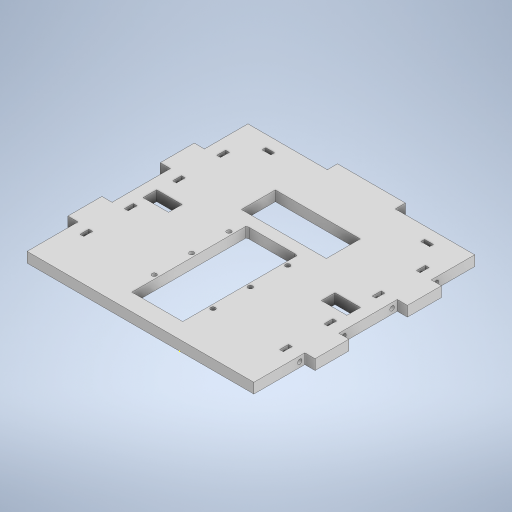
# Autodesk Inventor part: frame_upper1
Saved by Autodesk Inventor 2024 (Build 280153000, 153)
## iProperties
Created: 2024-09-07
Part Number: frame_upper1
Material: 일반
Document SubType Name: Modeling
Designer: jmha0
Density: 1 g/cm^3
Appearance: 기본값
Mass: 87.8648 g
Surface Area: 361.939 cm^2
Volume: 87.8648 cm^3
Author: jmha0
Autodesk Inventor part; units mm, degrees
(part 1 of 2)
ref_plane "YZ Plane" through (0, 0, 0) normal (1, 0, 0) x (0, 1, 0)
ref_plane "XZ Plane" through (0, 0, 0) normal (0, 1, 0) x (-1, 0, 0)
ref_plane "XY Plane" through (0, 0, 0) normal (0, 0, 1) x (1, 0, 0)
sketch "스케치1" plane through (0, 0, 0) normal (0, 1, 0) x (-1, 0, 0)
  line L0 (-51.929, 23.5866) -> (-51.929, -10.2551)
  line L1 (-51.929, -10.2551) -> (-45.929, -10.2551)
  line L2 (-45.929, -10.2551) -> (-45.929, -50.2551)
  line L3 (-45.929, -50.2551) -> (-51.929, -50.2551)
  line L4 (-51.929, -50.2551) -> (-51.929, -112.0968)
  line L5 (-51.929, -112.0968) -> (97.1074, -112.0968)
  line L6 (97.1074, -112.0968) -> (97.1074, -50.2551)
  line L7 (97.1074, -50.2551) -> (92.3803, -50.2551)
  line L8 (92.3803, -50.2551) -> (92.3803, -10.2551)
  line L9 (92.3803, -10.2551) -> (97.7439, -10.2551)
  line L10 (97.7439, -10.2551) -> (97.7439, 23.5866)
  line L11 (-51.929, 23.5866) -> (97.7439, 23.5866)
  line L12 (57.1074, -50.2551) -> (51.1074, -50.2551)
  line L13 (51.1074, -50.2551) -> (51.1074, -10.2551)
  line L14 (51.1074, -10.2551) -> (57.1074, -10.2551)
  line L15 (57.1074, -10.2551) -> (57.1074, -50.2551)
  line L16 (-5.2926, -50.2551) -> (-11.2926, -50.2551)
  line L17 (-11.2926, -50.2551) -> (-11.2926, -10.2551)
  line L18 (-11.2926, -10.2551) -> (-5.2926, -10.2551)
  line L19 (-5.2926, -10.2551) -> (-5.2926, -50.2551)
  circle A0 centre (40.2074, -56.8968) radius 1.45
  circle A1 centre (5.6074, -56.8968) radius 1.45
  circle A2 centre (40.2074, -34.8968) radius 1.45
  circle A3 centre (5.6074, -34.8968) radius 1.45
  circle A4 centre (40.2074, -12.8968) radius 1.45
  circle A5 centre (5.6074, -12.8968) radius 1.45
  line L20 (37.6074, 2.5866) -> (37.6074, -73.0968)
  line L21 (37.6074, -73.0968) -> (8.2074, -73.0968)
  line L22 (8.2074, -73.0968) -> (8.2074, 2.5866)
  line L23 (8.2074, 2.5866) -> (37.6074, 2.5866)
  line L24 (89.8574, 258.2156) -> (-43.6426, 258.2156)
  line L25 (-43.6426, 128.2156) -> (89.8574, 128.2156)
  arc A6 (3.3266, -10.6333) -> (2.8074, -12.3202) centre (5.8074, -12.3202) ccw
  line L26 (2.8074, -56.5734) -> (2.8074, -12.3202)
  arc A7 (2.8074, -56.5734) -> (3.3266, -58.2604) centre (5.8074, -56.5734) ccw
  line L27 (7.0145, -63.6837) -> (3.3266, -58.2604)
  arc A8 (7.0145, -63.6837) -> (9.4953, -64.9968) centre (9.4953, -61.9968) ccw
  line L28 (36.3195, -64.9968) -> (9.4953, -64.9968)
  arc A9 (36.3195, -64.9968) -> (38.8003, -63.6837) centre (36.3195, -61.9968) ccw
  line L29 (42.4882, -58.2604) -> (38.8003, -63.6837)
  arc A10 (42.4882, -58.2604) -> (43.0074, -56.5734) centre (40.0074, -56.5734) ccw
  line L30 (43.0074, -12.3202) -> (43.0074, -56.5734)
  arc A11 (43.0074, -12.3202) -> (42.4882, -10.6333) centre (40.0074, -12.3202) ccw
  line L31 (38.5027, -4.7722) -> (42.4882, -10.6333)
  arc A12 (38.5027, -4.7722) -> (36.8488, -3.8968) centre (36.8488, -5.8968) ccw
  line L32 (30.5574, -3.8968) -> (36.8488, -3.8968)
  arc A13 (32.0574, -5.3968) -> (30.5574, -3.8968) centre (30.5574, -5.3968) ccw
  line L33 (32.0574, -5.3968) -> (32.0574, -6.8968)
  arc A14 (32.0574, -6.8968) -> (34.4074, -9.2468) centre (34.4074, -6.8968) ccw
  line L34 (34.4074, -9.2468) -> (36.4074, -9.2468)
  arc A15 (37.4074, -10.2468) -> (36.4074, -9.2468) centre (36.4074, -10.2468) ccw
  line L35 (37.4074, -10.2468) -> (37.4074, -53.0468)
  arc A16 (36.4074, -54.0468) -> (37.4074, -53.0468) centre (36.4074, -53.0468) ccw
  line L36 (36.4074, -54.0468) -> (34.4074, -54.0468)
  arc A17 (34.4074, -54.0468) -> (32.0574, -56.3968) centre (34.4074, -56.3968) ccw
  line L37 (32.0574, -56.3968) -> (32.0574, -58.3968)
  arc A18 (31.0574, -59.3968) -> (32.0574, -58.3968) centre (31.0574, -58.3968) ccw
  line L38 (31.0574, -59.3968) -> (14.7574, -59.3968)
  arc A19 (13.7574, -58.3968) -> (14.7574, -59.3968) centre (14.7574, -58.3968) ccw
  line L39 (13.7574, -58.3968) -> (13.7574, -56.3968)
  arc A20 (13.7574, -56.3968) -> (11.4074, -54.0468) centre (11.4074, -56.3968) ccw
  line L40 (11.4074, -54.0468) -> (9.4074, -54.0468)
  arc A21 (8.4074, -53.0468) -> (9.4074, -54.0468) centre (9.4074, -53.0468) ccw
  line L41 (8.4074, -53.0468) -> (8.4074, -10.2468)
  arc A22 (9.4074, -9.2468) -> (8.4074, -10.2468) centre (9.4074, -10.2468) ccw
  line L42 (9.4074, -9.2468) -> (11.4074, -9.2468)
  arc A23 (11.4074, -9.2468) -> (13.7574, -6.8968) centre (11.4074, -6.8968) ccw
  line L43 (13.7574, -6.8968) -> (13.7574, -5.3968)
  arc A24 (15.2574, -3.8968) -> (13.7574, -5.3968) centre (15.2574, -5.3968) ccw
  line L44 (8.966, -3.8968) -> (15.2574, -3.8968)
  arc A25 (8.966, -3.8968) -> (7.3121, -4.7722) centre (8.966, -5.8968) ccw
  line L45 (3.3266, -10.6333) -> (7.3121, -4.7722)
  circle A26 centre (40.2074, -12.8968) radius 1.35
  circle A27 centre (40.2074, -34.8968) radius 1.35
  circle A28 centre (33.9074, -62.1968) radius 1.35
  circle A29 centre (5.6074, -12.8968) radius 1.35
  circle A30 centre (5.6074, -34.8968) radius 1.35
  circle A31 centre (11.9074, -62.1968) radius 1.35
  circle A32 centre (40.2074, -56.8968) radius 1.35
  circle A33 centre (5.6074, -56.8968) radius 1.35
  circle A34 centre (22.9074, -16.8968) radius 13.8
  circle A35 centre (22.9074, -27.8968) radius 1.2813
  circle A36 centre (30.6856, -24.675) radius 1.2813
  circle A37 centre (33.9074, -16.8968) radius 1.2813
  circle A38 centre (30.6856, -9.1186) radius 1.2813
  circle A39 centre (22.9074, -5.8968) radius 1.2813
  circle A40 centre (15.1292, -9.1186) radius 1.2813
  circle A41 centre (22.9074, -16.8968) radius 13.8
  circle A42 centre (22.9074, -16.8968) radius 7.2
  circle A43 centre (22.9074, -27.8968) radius 1.2813
  circle A44 centre (15.1292, -24.675) radius 1.2813
  circle A45 centre (11.9074, -16.8968) radius 1.2813
  circle A46 centre (15.1292, -9.1186) radius 1.2813
  circle A47 centre (22.9074, -5.8968) radius 1.2813
  circle A48 centre (30.6856, -9.1186) radius 1.2813
  circle A49 centre (33.9074, -16.8968) radius 1.2813
  circle A50 centre (30.6856, -24.675) radius 1.2813
  line L46 (23.1074, 258.2156) -> (23.1074, 238.2156)
  line L47 (23.2304, 248.2156) -> (38.2304, 248.2156)
  line L48 (38.2304, 248.2156) -> (8.2304, 248.2156)
  line L49 (8.2304, 248.2156) -> (8.2304, 173.2156)
  line L50 (8.2304, 173.2156) -> (38.2304, 173.2156)
  line L51 (38.2304, 173.2156) -> (38.2304, 248.2156)
  arc A51 (3.6496, 234.9792) -> (3.1304, 233.2922) centre (6.1304, 233.2922) ccw
  line L52 (3.1304, 189.039) -> (3.1304, 233.2922)
  arc A52 (3.1304, 189.039) -> (3.6496, 187.352) centre (6.1304, 189.039) ccw
  line L53 (7.3375, 181.9287) -> (3.6496, 187.352)
  arc A53 (7.3375, 181.9287) -> (9.8183, 180.6156) centre (9.8183, 183.6156) ccw
  line L54 (36.6425, 180.6156) -> (9.8183, 180.6156)
  arc A54 (36.6425, 180.6156) -> (39.1233, 181.9287) centre (36.6425, 183.6156) ccw
  line L55 (42.8112, 187.352) -> (39.1233, 181.9287)
  arc A55 (42.8112, 187.352) -> (43.3304, 189.039) centre (40.3304, 189.039) ccw
  line L56 (43.3304, 233.2922) -> (43.3304, 189.039)
  arc A56 (43.3304, 233.2922) -> (42.8112, 234.9792) centre (40.3304, 233.2922) ccw
  line L57 (38.8256, 240.8402) -> (42.8112, 234.9792)
  arc A57 (38.8256, 240.8402) -> (37.1718, 241.7156) centre (37.1718, 239.7156) ccw
  line L58 (30.8804, 241.7156) -> (37.1718, 241.7156)
  arc A58 (37.7304, 235.3656) -> (36.7304, 236.3656) centre (36.7304, 235.3656) ccw
  arc A59 (36.7304, 191.5656) -> (37.7304, 192.5656) centre (36.7304, 192.5656) ccw
  arc A60 (8.7304, 192.5656) -> (9.7304, 191.5656) centre (9.7304, 192.5656) ccw
  arc A61 (9.7304, 236.3656) -> (8.7304, 235.3656) centre (9.7304, 235.3656) ccw
  arc A62 (9.289, 241.7156) -> (7.6351, 240.8402) centre (9.289, 239.7156) ccw
  line L59 (3.6496, 234.9792) -> (7.6351, 240.8402)
  circle A63 centre (40.5304, 232.7156) radius 1.45
  circle A64 centre (40.5304, 210.7156) radius 1.45
  circle A65 centre (40.5304, 188.7156) radius 1.45
  circle A66 centre (5.9304, 188.7156) radius 1.45
  circle A67 centre (5.9304, 210.7156) radius 1.45
  circle A68 centre (5.9304, 232.7156) radius 1.45
  line L60 (41.9804, 210.7156) -> (49.8574, 210.7156)
  line L61 (89.8574, 180.7156) -> (89.8574, 220.7156)
  line L62 (-43.6426, 180.7156) -> (-43.6426, 220.7156)
  line L63 (-43.6426, 258.2156) -> (-43.6426, 128.2156)
  line L64 (89.8574, 128.2156) -> (89.8574, 258.2156)
  line L65 (8.2304, 258.2156) -> (8.2304, 248.2156)
  circle A69 centre (40.5304, 188.7156) radius 1.35
  circle A70 centre (40.5304, 210.7156) radius 1.35
  circle A71 centre (40.5304, 232.7156) radius 1.35
  circle A72 centre (5.9304, 232.7156) radius 1.35
  circle A73 centre (5.9304, 210.7156) radius 1.35
  circle A74 centre (5.9304, 188.7156) radius 1.35
  point P0 (0, 0)
  point P1 (54.2167, -116.1391)
  point P2 (22.9074, 23.5866)
  point P3 (22.9074, -16.8968)
  point P4 (38.2304, 181.0703)
  point P5 (8.2304, 181.0703)
  point P6 (8.2304, 241.4125)
  point P7 (38.2304, 241.4125)
  dimension "d0" = 149.0364
  dimension "d1" = 135.6834
  dimension "d4" = 21
  dimension "d5" = 20
  dimension "d6" = 29.4
  dimension "d7" = 75.6834
  dimension "d8" = 15
  dimension "d9" = 30
  dimension "d17" = 40
  dimension "d18" = 6
  dimension "d36" = 130
  dimension "d37" = 133.5
  dimension "d95" = 0.1
  dimension "d96" = 0.1
  dimension "d97" = 0.1
  dimension "d98" = 0.1
  dimension "d99" = 0.1
  dimension "d100" = 0.1
  constraints: 132 end point, 75 centre point, 64 point on circle, 3 horizontal, 3 parallel, 2 midpoint, 2 perpendicular, 2 vertical, 1 point on line
  measures "d0" distance between parallel lines of L6 L4
  measures "d1" distance between parallel lines of L5 L11
  measures "d4" distance from line of point (22.907, 23.587) L23
  measures "d5" distance of L46.end L46.start
  measures "d6" distance of L23.start L23.end
  measures "d7" distance of L23.end L21.start
  measures "d8" distance of L47.start L47.end
  measures "d9" distance of L50.end L49.end
  measures "d17" distance of L14.end L12.start
  measures "d18" distance of L12.start L12.end
  measures "d36" distance between parallel lines of L24 L25
  measures "d37" distance between parallel lines of L63 L64
  measures "d95" radial gap between concentric circles of A65 A69
  measures "d96" radial gap between concentric circles of A64 A70
  measures "d97" radial gap between concentric circles of A63 A71
  measures "d98" radial gap between concentric circles of A68 A72
  measures "d99" radial gap between concentric circles of A67 A73
  measures "d100" radial gap between concentric circles of A66 A74
extrude "돌출1" add sketch "스케치1" along normal blind 6 contours L64 L61 L25 L63 L62 L24 L65 L49 A62 L59 A51 L52 A52 L53 A53 L50 L51 A54 L55 A55 L56 A56 L57 A57 L47 L48 L46 | L46 L48 L65 L24 | L49 A53 L53 A52 L52 A51 L59 A62 | A53 L54 A54 L51 L50 L49 | A57 L57 A56 L56 A55 L55 A54 L51 | A63 | A64 | A65 | A66 | A67 | A68
sketch "스케치6" plane through (43.6426, 0, 258.2156) normal (1, 0, 0) x (0, 0, -1)
  line L0 (0, 0) -> (84.4, 0)
  line L1 (77.1453, 0) -> (10, 0) projected
  line L2 (0, 6) -> (130, 6) projected
  line L3 (84.4, 0) -> (104.4, 0)
  line L4 (104.4, 0) -> (104.4, 6)
  line L5 (104.4, 6) -> (84.4, 6)
  line L6 (84.4, 6) -> (84.4, 0)
  line L7 (0, 0) -> (130, 0) projected
  line L8 (0, 0) -> (130, 0) projected
  line L9 (130, 0) -> (130, 6) projected
  line L10 (0, 6) -> (130, 6) projected
  line L11 (0, 0) -> (0, 6) projected
  line L12 (89.4, 0) -> (99.4, 0)
  line L13 (99.4, 0) -> (99.4, 6)
  line L14 (99.4, 6) -> (89.4, 6)
  line L15 (89.4, 6) -> (89.4, 0)
  line L16 (89.4, 0) -> (99.4, 6) construction
  line L17 (99.4, 0) -> (89.4, 6) construction
  point P0 (258.2156, 0)
  point P1 (85, 0)
  point P2 (85, 0)
  point P3 (94.4, 3)
  dimension "d89" = 84.4
  dimension "d90" = 20
  dimension "d179" = 10
  constraints: 22 end point, 4 parallel, 3 point on line, 2 horizontal, 2 midpoint, 2 perpendicular
  measures "d89" distance of L0.start L0.end
  measures "d90" distance of L5.end L4.end
  measures "d179" distance of L14.end L13.end
extrude "돌출5" add sketch "스케치6" along normal blind 6 contours L2 L13 L3 L15
sketch "스케치7" plane through (-89.8574, 0, 128.2156) normal (-1, 0, 0) x (0, 0, 1)
  line L0 (25.6, 6) -> (25.6, 0) projected
  line L1 (0, 0) -> (130, 0) projected
  line L2 (130, 0) -> (130, 6) projected
  line L3 (0, 6) -> (130, 6) projected
  line L4 (0, 0) -> (0, 6) projected
  line L5 (45.6, 0) -> (45.6, 6) projected
  line L6 (0, 6) -> (130, 6) projected
  line L7 (0, 0) -> (130, 0) projected
  line L8 (25.6, 6) -> (35.6, 6)
  line L9 (30.6, 0) -> (40.6, 0)
  line L10 (40.6, 0) -> (40.6, 6)
  line L11 (40.6, 6) -> (30.6, 6)
  line L12 (30.6, 6) -> (30.6, 0)
  line L13 (30.6, 0) -> (40.6, 6) construction
  line L14 (40.6, 0) -> (30.6, 6) construction
  point P0 (-128.2156, 0)
  point P1 (35.6, 3)
  dimension "d180" = 10
  dimension "d181" = 10
  constraints: 14 end point, 2 midpoint, 2 parallel, 2 point on line, 1 horizontal, 1 perpendicular
  measures "d180" distance of L0.start L8.end
  measures "d181" distance of L11.end L10.end
extrude "돌출6" add sketch "스케치7" along normal blind 6 contours L3 L10 L1 L12
sketch "스케치8" plane through (43.6426, 0, 258.2156) normal (1, 0, 0) x (0, 0, -1)
  line L0 (0, 6) -> (89.4, 6) projected
  line L1 (0, 0) -> (0, 6) projected
  line L2 (0, 0) -> (89.4, 0) projected
  line L3 (0, 0) -> (89.4, 0) projected
  line L4 (130, 0) -> (130, 6) projected
  line L5 (99.4, 6) -> (130, 6) projected
  line L6 (104.4, 0) -> (110.4, 0)
  line L7 (110.4, 0) -> (110.4, 6)
  line L8 (110.4, 6) -> (104.4, 6)
  line L9 (104.4, 6) -> (104.4, 0)
  line L10 (84.4, 0) -> (78.4, 0)
  line L11 (78.4, 0) -> (78.4, 6)
  line L12 (78.4, 6) -> (84.4, 6)
  line L13 (84.4, 6) -> (84.4, 0)
  circle A0 centre (81.4, 3) radius 1.35
  circle A1 centre (107.4, 3) radius 1.35
  line L14 (99.4, 6) -> (99.4, 0) projected
  line L15 (99.4, 0) -> (130, 0) projected
  line L16 (89.4, 0) -> (89.4, 6) projected
  line L17 (0, 6) -> (89.4, 6) projected
  line L18 (0, 0) -> (0, 6) projected
  line L19 (99.4, 6) -> (99.4, 0) projected
  line L20 (99.4, 0) -> (130, 0) projected
  line L21 (130, 0) -> (130, 6) projected
  line L22 (99.4, 6) -> (130, 6) projected
  line L23 (89.4, 0) -> (89.4, 6) projected
  point P0 (258.2156, 0)
  dimension "d101" = 6
  dimension "d102" = 6
  dimension "d103" = 2.7
  dimension "d104" = 2.7
  constraints: 16 end point, 4 parallel, 2 centre point, 2 horizontal, 2 perpendicular, 2 point on line
  measures "d101" distance of L8.end L7.end
  measures "d102" distance of L11.end L12.end
  measures "d103" diameter of A0
  measures "d104" diameter of A1
extrude "돌출7" cut sketch "스케치8" against normal blind 16 contours A0 | A1
sketch "스케치9" plane through (-89.8574, 0, 128.2156) normal (-1, 0, 0) x (0, 0, 1)
  circle A0 centre (22.6, 3) radius 1.35 projected
  circle A1 centre (48.6, 3) radius 1.35 projected
  point P0 (-128.2156, 0)
extrude "돌출8" cut sketch "스케치9" against normal blind 16
sketch "스케치11" plane through (43.6426, 0, 128.2156) normal (0, 0, -1) x (-1, 0, 0)
  line L0 (0, 0) -> (133.5, 0) projected
  line L1 (133.5, 0) -> (133.5, 6) projected
  line L2 (0, 6) -> (133.5, 6) projected
  line L3 (0, 0) -> (0, 6) projected
  line L4 (0, 6) -> (20, 6)
  line L5 (133.5, 6) -> (113.5, 6)
  circle A0 centre (20, 3) radius 1.35
  circle A1 centre (113.5, 3) radius 1.35
  point P0 (43.6426, 0)
  dimension "d118" = 133.5
  dimension "d119" = 20
  dimension "d120" = 20
  dimension "d121" = 2.7
  dimension "d122" = 2.7
  constraints: 4 end point, 2 centre point, 2 point on line
  measures "d118" distance of L2.start L1.end
  measures "d119" distance of L2.start L4.end
  measures "d120" distance of L1.end L5.end
  measures "d121" diameter of A0
  measures "d122" diameter of A1
extrude "돌출10" cut sketch "스케치11" against normal blind 16 contours A0 | A1
sketch "스케치12" plane through (0, 6, 0) normal (0, 1, 0) x (1, 0, 0)
  line L0 (-71.2074, -144.2156) -> (-68.5074, -144.2156) projected
  line L1 (-71.2074, -144.2156) -> (-68.5074, -144.2156) projected
  line L2 (-71.2074, -128.2156) -> (-68.5074, -128.2156) projected
  line L3 (-71.2074, -144.2156) -> (-68.5074, -144.2156) projected
  line L4 (-71.2074, -128.2156) -> (-68.5074, -128.2156) projected
  line L5 (-89.8574, -152.1656) -> (-89.8574, -149.4656) projected
  line L6 (22.2926, -144.2156) -> (24.9926, -144.2156) projected
  line L7 (22.2926, -144.2156) -> (24.9926, -144.2156) projected
  line L8 (22.2926, -128.2156) -> (24.9926, -128.2156) projected
  line L9 (22.2926, -144.2156) -> (24.9926, -144.2156) projected
  line L10 (22.2926, -128.2156) -> (24.9926, -128.2156) projected
  line L11 (-89.8574, -152.1656) -> (-89.8574, -149.4656) projected
  line L12 (-89.8574, -128.2156) -> (-89.8574, -158.8156) projected
  line L13 (-89.8574, -128.2156) -> (-89.8574, -158.8156) projected
  line L14 (-89.8574, -128.2156) -> (-89.8574, -258.2156) projected
  line L15 (-89.8574, -128.2156) -> (-89.8574, -258.2156) projected
  line L16 (-83.8574, -148.2156) -> (-83.8574, -153.4156) projected
  line L17 (-83.8574, -153.4156) -> (-83.8574, -148.2156) projected
  line L18 (-83.8574, -153.4156) -> (-86.0574, -153.4156) projected
  line L19 (-86.0574, -153.4156) -> (-83.8574, -153.4156) projected
  line L20 (-86.0574, -153.4156) -> (-83.8574, -153.4156) projected
  line L21 (-83.8574, -153.4156) -> (-86.0574, -153.4156) projected
  line L22 (-89.8574, -152.1656) -> (-89.8574, -149.4656) projected
  line L23 (-86.0574, -152.1656) -> (-86.0574, -149.4656) projected
  line L24 (-86.0574, -148.2156) -> (-86.0574, -153.4156) projected
  line L25 (-83.8574, -148.2156) -> (-86.0574, -148.2156) projected
  line L26 (-83.8574, -148.2156) -> (-83.8574, -153.4156) projected
  line L27 (-83.8574, -153.4156) -> (-83.8574, -148.2156) projected
  line L28 (-86.0574, -152.1656) -> (-86.0574, -149.4656) projected
  line L29 (-86.0574, -153.4156) -> (-86.0574, -148.2156) projected
  line L30 (-86.0574, -148.2156) -> (-86.0574, -153.4156) projected
  line L31 (-86.0574, -148.2156) -> (-83.8574, -148.2156) projected
  line L32 (-83.8574, -148.2156) -> (-86.0574, -148.2156) projected
  line L33 (-86.0574, -148.2156) -> (-83.8574, -148.2156) projected
  line L34 (-86.0574, -153.4156) -> (-86.0574, -148.2156) projected
  line L35 (37.6426, -148.6131) -> (37.6426, -153.0181) projected
  line L36 (37.6426, -153.0181) -> (39.8426, -153.0181) projected
  line L37 (39.8426, -153.0181) -> (37.6426, -153.0181) projected
  line L38 (37.6426, -153.0181) -> (37.6426, -148.6131) projected
  line L39 (37.6426, -148.6131) -> (37.6426, -153.0181) projected
  line L40 (39.8426, -148.6131) -> (37.6426, -148.6131) projected
  line L41 (39.8426, -153.0181) -> (39.8426, -148.6131) projected
  line L42 (37.6426, -148.6131) -> (39.8426, -148.6131) projected
  line L43 (39.8426, -148.6131) -> (39.8426, -153.0181) projected
  line L44 (37.6426, -148.6131) -> (39.8426, -148.6131) projected
  line L45 (39.8426, -148.6131) -> (37.6426, -148.6131) projected
  line L46 (39.8426, -149.4656) -> (39.8426, -152.1656) projected
  line L47 (39.8426, -148.6131) -> (39.8426, -153.0181) projected
  line L48 (39.8426, -153.0181) -> (39.8426, -148.6131) projected
  line L49 (39.8426, -153.0181) -> (37.6426, -153.0181) projected
  line L50 (37.6426, -153.0181) -> (39.8426, -153.0181) projected
  line L51 (24.9926, -128.2156) -> (24.9926, -144.2156) projected
  line L52 (22.2926, -128.2156) -> (22.2926, -144.2156) projected
  line L53 (-68.5074, -128.2156) -> (-68.5074, -144.2156) projected
  line L54 (-71.2074, -128.2156) -> (-71.2074, -144.2156) projected
  line L55 (23.6426, -144.2156) -> (23.6426, -143.1156)
  line L56 (43.6426, -128.2156) -> (-89.8574, -128.2156) projected
  line L57 (43.6426, -128.2156) -> (-89.8574, -128.2156) projected
  line L58 (-71.2074, -128.2156) -> (-68.5074, -128.2156) projected
  line L59 (22.2926, -128.2156) -> (24.9926, -128.2156) projected
  line L60 (43.6426, -128.2156) -> (-89.8574, -128.2156) projected
  line L61 (43.6426, -128.2156) -> (-89.8574, -128.2156) projected
  line L62 (43.6426, -158.8156) -> (43.6426, -128.2156) projected
  line L63 (43.6426, -258.2156) -> (43.6426, -128.2156) projected
  line L64 (49.6426, -168.8156) -> (49.6426, -158.8156) projected
  line L65 (49.6426, -158.8156) -> (49.6426, -168.8156) projected
  line L66 (43.6426, -153.8156) -> (49.6426, -153.8156) projected
  line L67 (43.6426, -173.8156) -> (49.6426, -173.8156) projected
  line L68 (43.6426, -173.8156) -> (49.6426, -173.8156) projected
  line L69 (22.2926, -144.2156) -> (24.9926, -144.2156) projected
  line L70 (43.6426, -173.8156) -> (49.6426, -173.8156) projected
  line L71 (43.6426, -173.8156) -> (49.6426, -173.8156) projected
  line L72 (22.2926, -144.2156) -> (24.9926, -144.2156) projected
  line L73 (22.2926, -128.2156) -> (24.9926, -128.2156) projected
  line L74 (49.6426, -158.8156) -> (49.6426, -168.8156) projected
  line L75 (49.6426, -168.8156) -> (49.6426, -158.8156) projected
  line L76 (43.6426, -153.8156) -> (49.6426, -153.8156) projected
  line L77 (43.6426, -153.8156) -> (49.6426, -153.8156) projected
  line L78 (43.6426, -153.8156) -> (49.6426, -153.8156) projected
  line L79 (43.6426, -149.4656) -> (43.6426, -152.1656) projected
  line L80 (27.6426, -149.4656) -> (27.6426, -152.1656) projected
  line L81 (27.6426, -149.4656) -> (27.6426, -152.1656) projected
  line L82 (27.6426, -149.4656) -> (27.6426, -152.1656) projected
  line L83 (43.6426, -149.4656) -> (43.6426, -152.1656) projected
  line L84 (43.6426, -149.4656) -> (43.6426, -152.1656) projected
  line L85 (43.6426, -258.2156) -> (43.6426, -168.8156) projected
  line L86 (43.6426, -158.8156) -> (43.6426, -128.2156) projected
  line L87 (-95.8574, -168.8156) -> (-95.8574, -158.8156) projected
  line L88 (-95.8574, -158.8156) -> (-95.8574, -168.8156) projected
  line L89 (-89.8574, -153.8156) -> (-95.8574, -153.8156) projected
  line L90 (-89.8574, -153.8156) -> (-95.8574, -153.8156) projected
  line L91 (-89.8574, -173.8156) -> (-95.8574, -173.8156) projected
  line L92 (-89.8574, -173.8156) -> (-95.8574, -173.8156) projected
  line L93 (-73.8574, -152.1656) -> (-73.8574, -149.4656) projected
  line L94 (-73.8574, -152.1656) -> (-73.8574, -149.4656) projected
  line L95 (-89.8574, -173.8156) -> (-95.8574, -173.8156) projected
  line L96 (-89.8574, -173.8156) -> (-95.8574, -173.8156) projected
  line L97 (-95.8574, -158.8156) -> (-95.8574, -168.8156) projected
  line L98 (-95.8574, -168.8156) -> (-95.8574, -158.8156) projected
  line L99 (-73.8574, -152.1656) -> (-73.8574, -149.4656) projected
  line L100 (-89.8574, -152.1656) -> (-89.8574, -149.4656) projected
  line L101 (-71.2074, -144.2156) -> (-68.5074, -144.2156) projected
  line L102 (-71.2074, -128.2156) -> (-68.5074, -128.2156) projected
  line L103 (-89.8574, -152.1656) -> (-89.8574, -149.4656) projected
  line L104 (-89.8574, -128.2156) -> (-89.8574, -158.8156) projected
  line L105 (-89.8574, -128.2156) -> (-89.8574, -158.8156) projected
  line L106 (-89.8574, -153.8156) -> (-95.8574, -153.8156) projected
  line L107 (-89.8574, -153.8156) -> (-95.8574, -153.8156) projected
  line L108 (-71.2074, -144.2156) -> (-68.5074, -144.2156) projected
  line L109 (43.6426, -149.4656) -> (27.6426, -149.4656) projected
  line L110 (43.6426, -152.1656) -> (27.6426, -152.1656) projected
  line L111 (-89.8574, -149.4656) -> (-73.8574, -149.4656) projected
  line L112 (-89.8574, -152.1656) -> (-73.8574, -152.1656) projected
  line L113 (34.5426, -148.2156) -> (36.7426, -148.2156)
  line L114 (36.7426, -148.2156) -> (36.7426, -153.4156)
  line L115 (36.7426, -153.4156) -> (34.5426, -153.4156)
  line L116 (34.5426, -153.4156) -> (34.5426, -148.2156)
  line L117 (34.5426, -148.2156) -> (36.7426, -153.4156) construction
  line L118 (36.7426, -148.2156) -> (34.5426, -153.4156) construction
  line L119 (21.0426, -135.1156) -> (26.2426, -135.1156)
  line L120 (26.2426, -135.1156) -> (26.2426, -137.3156)
  line L121 (26.2426, -137.3156) -> (21.0426, -137.3156)
  line L122 (21.0426, -137.3156) -> (21.0426, -135.1156)
  line L123 (21.0426, -135.1156) -> (26.2426, -137.3156) construction
  line L124 (26.2426, -135.1156) -> (21.0426, -137.3156) construction
  line L125 (-72.4574, -135.1156) -> (-67.2574, -135.1156)
  line L126 (-67.2574, -135.1156) -> (-67.2574, -137.3156)
  line L127 (-67.2574, -137.3156) -> (-72.4574, -137.3156)
  line L128 (-72.4574, -137.3156) -> (-72.4574, -135.1156)
  line L129 (-72.4574, -135.1156) -> (-67.2574, -137.3156) construction
  line L130 (-67.2574, -135.1156) -> (-72.4574, -137.3156) construction
  line L131 (-82.9574, -148.2156) -> (-80.7574, -148.2156)
  line L132 (-80.7574, -148.2156) -> (-80.7574, -153.4156)
  line L133 (-80.7574, -153.4156) -> (-82.9574, -153.4156)
  line L134 (-82.9574, -153.4156) -> (-82.9574, -148.2156)
  line L135 (-82.9574, -148.2156) -> (-80.7574, -153.4156) construction
  line L136 (-80.7574, -148.2156) -> (-82.9574, -153.4156) construction
  circle A0 centre (-40.5304, -188.7156) radius 1.35 projected
  circle A1 centre (-40.5304, -188.7156) radius 1.35 projected
  circle A2 centre (-40.5304, -188.7156) radius 1.35 projected
  arc A3 (-36.6425, -180.6156) -> (-38.2304, -181.0703) centre (-36.6425, -183.6156) ccw projected
  line L137 (-36.6425, -180.6156) -> (-9.8183, -180.6156) projected
  line L138 (-36.6425, -180.6156) -> (-9.8183, -180.6156) projected
  line L139 (-36.6425, -180.6156) -> (-9.8183, -180.6156) projected
  line L140 (-36.6425, -180.6156) -> (-9.8183, -180.6156) projected
  circle A4 centre (-5.9304, -188.7156) radius 1.35 projected
  circle A5 centre (-5.9304, -188.7156) radius 1.35 projected
  circle A6 centre (-5.9304, -188.7156) radius 1.35 projected
  circle A7 centre (-5.9304, -188.7156) radius 1.35 projected
  arc A8 (-36.6425, -180.6156) -> (-38.2304, -181.0703) centre (-36.6425, -183.6156) ccw projected
  arc A9 (-8.2304, -181.0703) -> (-9.8183, -180.6156) centre (-9.8183, -183.6156) ccw projected
  arc A10 (-8.2304, -181.0703) -> (-9.8183, -180.6156) centre (-9.8183, -183.6156) ccw projected
  arc A11 (-8.2304, -181.0703) -> (-9.8183, -180.6156) centre (-9.8183, -183.6156) ccw projected
  arc A12 (-8.2304, -181.0703) -> (-9.8183, -180.6156) centre (-9.8183, -183.6156) ccw projected
  arc A13 (-36.6425, -180.6156) -> (-38.2304, -181.0703) centre (-36.6425, -183.6156) ccw projected
  arc A14 (-36.6425, -180.6156) -> (-38.2304, -181.0703) centre (-36.6425, -183.6156) ccw projected
  line L141 (-73.8574, -178.1656) -> (-73.8574, -175.4656) projected
  line L142 (-73.8574, -178.1656) -> (-73.8574, -175.4656) projected
  line L143 (-73.8574, -178.1656) -> (-73.8574, -175.4656) projected
  line L144 (-89.8574, -178.1656) -> (-89.8574, -175.4656) projected
  circle A15 centre (-40.5304, -188.7156) radius 1.35 projected
  line L145 (-89.8574, -178.1656) -> (-89.8574, -175.4656) projected
  line L146 (43.6426, -175.4656) -> (43.6426, -178.1656) projected
  line L147 (27.6426, -175.4656) -> (27.6426, -178.1656) projected
  line L148 (27.6426, -175.4656) -> (27.6426, -178.1656) projected
  line L149 (27.6426, -175.4656) -> (27.6426, -178.1656) projected
  line L150 (43.6426, -175.4656) -> (43.6426, -178.1656) projected
  line L151 (43.6426, -173.8156) -> (49.6426, -173.8156) projected
  line L152 (43.6426, -173.8156) -> (49.6426, -173.8156) projected
  line L153 (-89.8574, -173.8156) -> (-95.8574, -173.8156) projected
  line L154 (-89.8574, -173.8156) -> (-95.8574, -173.8156) projected
  line L155 (-89.8574, -175.4656) -> (-73.8574, -175.4656) projected
  line L156 (-89.8574, -178.1656) -> (-73.8574, -178.1656) projected
  line L157 (43.6426, -175.4656) -> (27.6426, -175.4656) projected
  line L158 (43.6426, -178.1656) -> (27.6426, -178.1656) projected
  line L159 (-82.9574, -179.4156) -> (-80.7574, -179.4156)
  line L160 (-80.7574, -179.4156) -> (-80.7574, -174.2156)
  line L161 (-80.7574, -174.2156) -> (-82.9574, -174.2156)
  line L162 (-82.9574, -174.2156) -> (-82.9574, -179.4156)
  line L163 (-82.9574, -179.4156) -> (-80.7574, -174.2156) construction
  line L164 (-80.7574, -179.4156) -> (-82.9574, -174.2156) construction
  line L165 (34.5426, -179.4156) -> (36.7426, -179.4156)
  line L166 (36.7426, -179.4156) -> (36.7426, -174.2156)
  line L167 (36.7426, -174.2156) -> (34.5426, -174.2156)
  line L168 (34.5426, -174.2156) -> (34.5426, -179.4156)
  line L169 (34.5426, -179.4156) -> (36.7426, -174.2156) construction
  line L170 (36.7426, -179.4156) -> (34.5426, -174.2156) construction
  line L171 (43.6426, -158.8156) -> (43.6426, -128.2156) projected
  line L172 (43.6426, -258.2156) -> (43.6426, -168.8156) projected
  line L173 (-89.8574, -168.8156) -> (-89.8574, -258.2156) projected
  line L174 (-89.8574, -168.8156) -> (-89.8574, -258.2156) projected
  line L175 (-89.8574, -168.8156) -> (-89.8574, -258.2156) projected
  line L176 (-89.8574, -168.8156) -> (-89.8574, -258.2156) projected
  point P0 (0, 0)
  point P1 (35.6426, -150.8156)
  point P2 (23.6426, -136.2156)
  point P3 (-69.8574, -136.2156)
  point P4 (-81.8574, -150.8156)
  point P5 (-81.8574, -176.8156)
  point P6 (35.6426, -176.8156)
  dimension "d125" = 1.1
  dimension "d126" = 2.2
  dimension "d127" = 5.2
  dimension "d128" = 5.2
  dimension "d129" = 2.2
  dimension "d130" = 5.2
  dimension "d131" = 2.2
  dimension "d166" = 5.2
  dimension "d167" = 2.2
  constraints: 74 end point, 13 midpoint, 12 parallel, 6 horizontal, 6 perpendicular, 1 point on line, 1 vertical, 11 other
  measures "d125" distance of L55.start L55.end
  measures "d126" distance of L114.end L115.end
  measures "d127" distance of L113.end L114.end
  measures "d128" distance of L120.end L121.end
  measures "d129" distance of L119.end L120.end
  measures "d130" distance of L126.end L127.end
  measures "d131" distance of L132.end L133.end
  measures "d166" distance of L160.end L159.end
  measures "d167" distance of L167.end L166.end
extrude "돌출11" cut sketch "스케치12" against normal blind 16 contours L127 L128 L125 L54 | L54 L125 L53 L127 | L53 L125 L126 L127 | L134 L111 L132 L112 | L112 L132 L133 L134 | L134 L131 L132 L111 | L121 L122 L119 L52 | L52 L119 L51 L121 | L51 L119 L120 L121 | L162 L161 L160 L155 | L155 L160 L156 L162 | L156 L160 L159 L162 | L114 L110 L116 L109 | L109 L116 L113 L114 | L114 L115 L116 L110 | L166 L165 L168 L158 | L158 L168 L157 L166 | L157 L168 L167 L166
sketch "스케치13" plane through (0, 6, 0) normal (0, 1, 0) x (1, 0, 0)
  line L0 (-67.2574, -135.1156) -> (-67.2574, -137.3156) projected
  line L1 (-67.2574, -137.3156) -> (-72.4574, -137.3156) projected
  line L2 (-72.4574, -137.3156) -> (-72.4574, -135.1156) projected
  line L3 (-72.4574, -135.1156) -> (-67.2574, -135.1156) projected
  line L4 (21.0426, -135.1156) -> (26.2426, -135.1156) projected
  line L5 (26.2426, -135.1156) -> (26.2426, -137.3156) projected
  line L6 (26.2426, -137.3156) -> (21.0426, -137.3156) projected
  line L7 (21.0426, -137.3156) -> (21.0426, -135.1156) projected
  line L8 (-80.7574, -148.2156) -> (-80.7574, -153.4156) projected
  line L9 (-80.7574, -153.4156) -> (-82.9574, -153.4156) projected
  line L10 (-82.9574, -153.4156) -> (-82.9574, -148.2156) projected
  line L11 (-82.9574, -148.2156) -> (-80.7574, -148.2156) projected
  line L12 (34.5426, -148.2156) -> (36.7426, -148.2156) projected
  line L13 (36.7426, -148.2156) -> (36.7426, -153.4156) projected
  line L14 (36.7426, -153.4156) -> (34.5426, -153.4156) projected
  line L15 (34.5426, -153.4156) -> (34.5426, -148.2156) projected
  line L16 (-8.2304, -181.0703) -> (-8.2304, -248.2156) projected
  line L17 (-8.2304, -248.2156) -> (-38.2304, -248.2156) projected
  line L18 (-38.2304, -248.2156) -> (-38.2304, -181.0703) projected
  arc A0 (-36.6425, -180.6156) -> (-38.2304, -181.0703) centre (-36.6425, -183.6156) ccw projected
  line L19 (-36.6425, -180.6156) -> (-9.8183, -180.6156) projected
  arc A1 (-8.2304, -181.0703) -> (-9.8183, -180.6156) centre (-9.8183, -183.6156) ccw projected
  line L20 (43.6426, -258.2156) -> (43.6426, -168.8156) projected
  line L21 (49.6426, -158.8156) -> (49.6426, -168.8156) projected
  line L22 (43.6426, -158.8156) -> (43.6426, -128.2156) projected
  line L23 (43.6426, -128.2156) -> (-89.8574, -128.2156) projected
  line L24 (-89.8574, -128.2156) -> (-89.8574, -158.8156) projected
  line L25 (-89.8574, -258.2156) -> (43.6426, -258.2156) projected
  circle A2 centre (-5.9304, -232.7156) radius 1.35 projected
  circle A3 centre (-5.9304, -210.7156) radius 1.35 projected
  circle A4 centre (-5.9304, -188.7156) radius 1.35 projected
  circle A5 centre (-40.5304, -188.7156) radius 1.35 projected
  circle A6 centre (-40.5304, -232.7156) radius 1.35 projected
  circle A7 centre (-40.5304, -210.7156) radius 1.35 projected
  line L26 (-53.1074, -153.8156) -> (6.8926, -153.8156)
  line L27 (6.8926, -153.8156) -> (6.8926, -173.8156)
  line L28 (6.8926, -173.8156) -> (-53.1074, -173.8156)
  line L29 (-53.1074, -173.8156) -> (-53.1074, -153.8156)
  line L30 (-53.1074, -153.8156) -> (6.8926, -173.8156) construction
  line L31 (6.8926, -153.8156) -> (-53.1074, -173.8156) construction
  line L32 (-48.1074, -153.8156) -> (1.8926, -153.8156)
  line L33 (1.8926, -153.8156) -> (1.8926, -173.8156)
  line L34 (1.8926, -173.8156) -> (-48.1074, -173.8156)
  line L35 (-48.1074, -173.8156) -> (-48.1074, -153.8156)
  line L36 (-48.1074, -153.8156) -> (1.8926, -173.8156) construction
  line L37 (1.8926, -153.8156) -> (-48.1074, -173.8156) construction
  line L38 (43.6426, -168.8156) -> (49.6426, -168.8156) projected
  line L39 (43.6426, -158.8156) -> (49.6426, -158.8156) projected
  line L40 (-89.8574, -158.8156) -> (-95.8574, -158.8156) projected
  line L41 (-95.8574, -168.8156) -> (-95.8574, -158.8156) projected
  line L42 (-89.8574, -168.8156) -> (-95.8574, -168.8156) projected
  line L43 (-89.8574, -168.8156) -> (-89.8574, -258.2156) projected
  point P0 (0, 0)
  point P1 (-23.1074, -163.8156)
  dimension "d134" = 60
  dimension "d137" = 50
  constraints: 24 end point, 4 midpoint, 4 parallel, 2 horizontal, 2 perpendicular, 1 point on line
  measures "d134" distance of L27.end L28.end
  measures "d137" distance of L33.end L34.end
extrude "돌출12" cut sketch "스케치13" against normal blind 16 contours L26 L33 L28 L35
sketch "스케치14" plane through (-89.8574, 0, 258.2156) normal (0, 0, 1) x (1, 0, 0)
  point P0 (89.8574, 0)
sketch "스케치15" plane through (43.6426, 0, 128.2156) normal (0, 0, -1) x (-1, 0, 0)
  circle A0 centre (113.5, 3) radius 1.35 projected
  circle A1 centre (20, 3) radius 1.35 projected
  line L0 (0, 0) -> (133.5, 0) projected
  line L1 (133.5, 0) -> (133.5, 6) projected
  line L2 (0, 6) -> (133.5, 6) projected
  line L3 (0, 0) -> (0, 6) projected
  line L4 (46.75, 0) -> (86.75, 0)
  line L5 (86.75, 0) -> (86.75, 6)
  line L6 (86.75, 6) -> (46.75, 6)
  line L7 (46.75, 6) -> (46.75, 0)
  line L8 (46.75, 0) -> (86.75, 6) construction
  line L9 (86.75, 0) -> (46.75, 6) construction
  point P0 (43.6426, 0)
  point P1 (66.75, 3)
  dimension "d138" = 40
  constraints: 12 end point, 2 midpoint, 2 parallel, 1 horizontal, 1 perpendicular, 1 point on line
  measures "d138" distance of L6.end L5.end
extrude "돌출13" add sketch "스케치15" along normal blind 6 contours L7 L2 L5 L0
sketch "스케치16" plane through (43.6426, 0, 258.2156) normal (1, 0, 0) x (0, 0, -1)
  circle A0 centre (81.4, 3) radius 1.35 projected
  line L0 (0, 6) -> (89.4, 6) projected
  line L1 (0, 0) -> (0, 6) projected
  line L2 (0, 0) -> (89.4, 0) projected
  line L3 (99.4, 6) -> (89.4, 6) projected
  line L4 (89.4, 0) -> (99.4, 0) projected
  line L5 (123.1, 6) -> (123.1, 0) projected
  line L6 (130, 0) -> (130, 6) projected
  line L7 (130, 0) -> (136, 0) projected
  line L8 (136, 6) -> (136, 0) projected
  line L9 (130, 6) -> (136, 6) projected
  circle A1 centre (107.4, 3) radius 1.35 projected
  line L10 (0, 0) -> (89.4, 0) projected
  line L11 (130, 0) -> (130, 6) projected
  line L12 (99.4, 6) -> (130, 6) projected
  line L13 (0, 6) -> (40, 6)
  line L14 (50, 0) -> (50, 6)
  line L15 (50, 6) -> (30, 6)
  line L16 (30, 6) -> (30, 0)
  line L17 (30, 0) -> (50, 0)
  line L18 (50, 0) -> (30, 6) construction
  line L19 (50, 6) -> (30, 0) construction
  line L20 (35, 0) -> (45, 0)
  line L21 (45, 0) -> (45, 6)
  line L22 (45, 6) -> (35, 6)
  line L23 (35, 6) -> (35, 0)
  line L24 (35, 0) -> (45, 6) construction
  line L25 (45, 0) -> (35, 6) construction
  line L26 (89.4, 0) -> (99.4, 0)
  line L27 (99.4, 0) -> (99.4, 6)
  line L28 (99.4, 6) -> (89.4, 6)
  line L29 (89.4, 6) -> (89.4, 0)
  line L30 (89.4, 0) -> (99.4, 6) construction
  line L31 (99.4, 0) -> (89.4, 6) construction
  line L32 (99.4, 6) -> (99.4, 0) projected
  line L33 (99.4, 0) -> (130, 0) projected
  line L34 (130, 0) -> (130, 6) projected
  line L35 (99.4, 6) -> (130, 6) projected
  line L36 (89.4, 0) -> (89.4, 6) projected
  line L37 (99.4, 0) -> (99.4, 6) projected
  line L38 (89.4, 6) -> (89.4, 0) projected
  line L39 (99.4, 6) -> (99.4, 0) projected
  line L40 (99.4, 0) -> (130, 0) projected
  line L41 (89.4, 0) -> (89.4, 6) projected
  line L42 (0, 6) -> (89.4, 6) projected
  line L43 (0, 0) -> (0, 6) projected
  point P0 (258.2156, 0)
  point P1 (40, 3)
  point P2 (94.4, 3)
  dimension "d141" = 40
  dimension "d142" = 20
  dimension "d177" = 10
  dimension "d178" = 10
  constraints: 38 end point, 6 midpoint, 6 parallel, 4 perpendicular, 3 point on line, 2 horizontal
  measures "d141" distance of L0.start L13.end
  measures "d142" distance of L15.end L14.end
  measures "d177" distance of L22.end L21.end
  measures "d178" distance of L28.end L27.end
extrude "돌출14" add sketch "스케치16" along normal blind 6 contours L0 L21 L2 L23
sketch "스케치17" plane through (-89.8574, 0, 258.2156) normal (-1, 0, 0) x (0, 0, 1)
  line L0 (-24.15, 6) -> (-24.15, 0) projected
  line L1 (-26.85, 6) -> (-26.85, 0) projected
  line L2 (-50, 6) -> (-50, 0) projected
  line L3 (-48.85, 6) -> (-48.85, 0) projected
  line L4 (-46.15, 6) -> (-46.15, 0) projected
  line L5 (-30, 0) -> (-30, 6) projected
  line L6 (-50, 6) -> (-30, 6)
  line L7 (-30, 6) -> (-30, 0)
  line L8 (-30, 0) -> (-50, 0)
  line L9 (-50, 0) -> (-50, 6)
  line L10 (-89.4, 6) -> (0, 6) projected
  circle A0 centre (-81.4, 3) radius 1.35 projected
  line L11 (-89.4, 6) -> (-89.4, 0) projected
  line L12 (-89.4, 0) -> (0, 0) projected
  line L13 (0, 0) -> (0, 6) projected
  line L14 (-89.4, 6) -> (0, 6) projected
  line L15 (-35, 0) -> (-35, 6) projected
  line L16 (-45, 0) -> (-35, 0)
  line L17 (-35, 0) -> (-35, 6)
  line L18 (-35, 6) -> (-45, 6)
  line L19 (-45, 6) -> (-45, 0)
  line L20 (-45, 0) -> (-35, 6) construction
  line L21 (-35, 0) -> (-45, 6) construction
  point P0 (-258.2156, 0)
  point P1 (-40, 3)
  dimension "d182" = 10
  constraints: 20 end point, 4 parallel, 2 horizontal, 2 midpoint, 2 perpendicular, 1 other
  measures "d182" distance of L18.end L15.end
extrude "돌출15" add sketch "스케치17" along normal blind 6 contours L15 L8 L19 L6
sketch "스케치18" plane through (-89.8574, 0, 173.8156) normal (-1, 0, 0) x (0, 0, 1)
  circle A0 centre (3, 3) radius 1.35 projected
  line L0 (-5, 6) -> (39.4, 6) projected
  line L1 (-5, 0) -> (39.4, 0) projected
  line L2 (-45.6, 0) -> (-15, 0) projected
  line L3 (84.4, 0) -> (84.4, 6) projected
  line L4 (49.4, 6) -> (84.4, 6) projected
  line L5 (34.4, 6) -> (31.4, 6)
  line L6 (49.4, 6) -> (39.4, 6) projected
  line L7 (39.4, 0) -> (49.4, 0) projected
  circle A1 centre (31.4, 3) radius 1.35
  line L8 (54.4, 3) -> (57.4, 3)
  circle A2 centre (57.4, 3) radius 1.35
  line L9 (-45.6, 0) -> (-15, 0) projected
  line L10 (84.4, 0) -> (84.4, 6) projected
  line L11 (49.4, 6) -> (84.4, 6) projected
  line L12 (-45.6, 0) -> (-45.6, 6) projected
  line L13 (-15, 0) -> (-15, 6) projected
  line L14 (-45.6, 6) -> (-15, 6) projected
  line L15 (-5, 6) -> (-5, 0) projected
  line L16 (49.4, 0) -> (84.4, 0) projected
  line L17 (49.4, 0) -> (49.4, 6) projected
  line L18 (39.4, 6) -> (39.4, 0) projected
  line L19 (-15, 0) -> (-15, 6) projected
  line L20 (-45.6, 6) -> (-15, 6) projected
  line L21 (-45.6, 0) -> (-45.6, 6) projected
  line L22 (49.4, 6) -> (49.4, 0) projected
  line L23 (49.4, 0) -> (84.4, 0) projected
  line L24 (39.4, 0) -> (39.4, 6) projected
  line L25 (-5, 6) -> (39.4, 6) projected
  line L26 (-5, 6) -> (-5, 0) projected
  line L27 (-5, 0) -> (39.4, 0) projected
  line L28 (49.4, 6) -> (49.4, 0) projected
  line L29 (39.4, 0) -> (39.4, 6) projected
  point P0 (-173.8156, 0)
  dimension "d147" = 3
  dimension "d148" = 2.7
  dimension "d149" = 3
  dimension "d150" = 2.7
  constraints: 4 end point, 2 centre point, 1 coincident, 1 horizontal, 1 point on line
  measures "d147" distance of L5.start L5.end
  measures "d148" diameter of A1
  measures "d149" distance of L8.start L8.end
  measures "d150" diameter of A2
extrude "돌출16" cut sketch "스케치18" against normal blind 16 contours A1 | A2
sketch "스케치19" plane through (43.6426, 0, 258.2156) normal (1, 0, 0) x (0, 0, -1)
  circle A0 centre (27, 3) radius 1.35 projected
  circle A1 centre (53, 3) radius 1.35 projected
  point P0 (258.2156, 0)
extrude "돌출17" cut sketch "스케치19" against normal blind 16